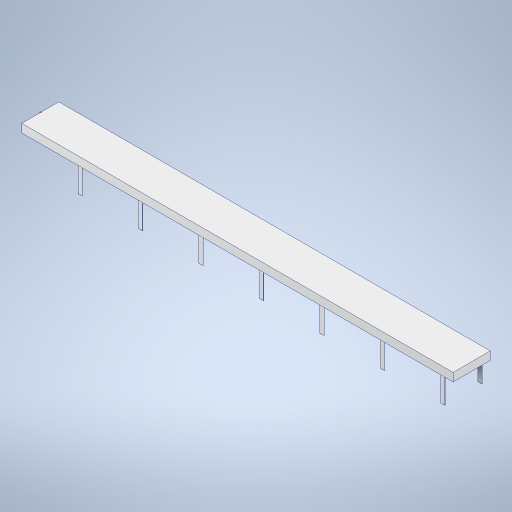
# Autodesk Inventor part: CableTray
Saved by Autodesk Inventor 2023.1 (Build 271208000, 208)
## iProperties
Created: 2023-06-07
Part Number: CableTray
Material: Aluminum 6061
Document SubType Name: Modeling
Designer: rwc6
Density: 2.7 g/cm^3
Appearance: Aluminum - Flat
tray_h: 4.000 in
tray_w: 18.000 in
leg_e: 11.811 in
Author: rwc6
Autodesk Inventor part; units mm, degrees
ref_plane "YZ Plane" through (0, 0, 0) normal (1, 0, 0) x (0, 1, 0)
ref_plane "XZ Plane" through (0, 0, 0) normal (0, 1, 0) x (-1, 0, 0)
ref_plane "XY Plane" through (0, 0, 0) normal (0, 0, 1) x (1, 0, 0)
sketch "Sketch1" plane through (0, 0, 0) normal (1, 0, 0) x (0, 1, 0)
  line L0 (50.8, 228.6) -> (-50.8, 228.6)
  line L1 (-50.8, 228.6) -> (-50.8, -228.6)
  line L2 (-50.8, -228.6) -> (50.8, -228.6)
  line L3 (50.8, -228.6) -> (50.8, 228.6)
  line L4 (50.8, 228.6) -> (-50.8, -228.6) construction
  line L5 (-50.8, 228.6) -> (50.8, -228.6) construction
  point P0 (0, 0)
  dimension "d0" = 101.6
  dimension "d1" = 457.2
  constraints: 12 end point, 2 midpoint, 2 parallel, 1 horizontal, 1 perpendicular
  measures "d0" distance of L2.end L1.end
  measures "d1" distance of L1.end L0.end
extrude "Extrusion1" add sketch "Sketch1" along normal blind 5300
sketch "Sketch2" plane through (0, -50.8, -228.6) normal (0, -1, 0) x (1, 0, 0)
  line L0 (5200, 457.2) -> (5149.2, 457.2)
  line L1 (5149.2, 457.2) -> (5149.2, 455.6125)
  line L2 (5149.2, 455.6125) -> (5200, 455.6125)
  line L3 (5200, 455.6125) -> (5200, 457.2)
  line L4 (5300, 457.2) -> (5300, 0) projected
  line L5 (0, 457.2) -> (5300, 457.2) projected
  point P0 (0, 228.6)
  dimension "d4" = 100
  dimension "d5" = 0
  dimension "d6" = 1.5875
  dimension "d7" = 50.8
  constraints: 8 end point, 2 parallel, 1 horizontal, 1 perpendicular
  measures "d4" distance between parallel lines of L4 L3
  measures "d5" distance between parallel lines of L5 L0
  measures "d6" distance between parallel lines of L2 L0
  measures "d7" distance between parallel lines of L3 L1
extrude "Extrusion2" add sketch "Sketch2" along normal blind 300
pattern_linear "Rectangular Pattern1" count 2 spacing 455.6125 along (0, 0, -1) count 7 spacing 742.9 along (-1, 0, 0) of "Extrusion2"
equation "\"d0\" = tray_h"
equation "\"d1\" = tray_w"
equation "\"d2\" = tray_e"
equation "\"d6\" = leg_w"
equation "\"d7\" = leg_h"
equation "\"d8\" = leg_e"
equation "\"tray_h\" = 101.6"
equation "\"tray_w\" = 457.2"
equation "\"tray_e\" = 5300"
equation "\"leg_h\" = 50.8"
equation "\"leg_w\" = 1.5875"
equation "\"leg_e\" = 300"
